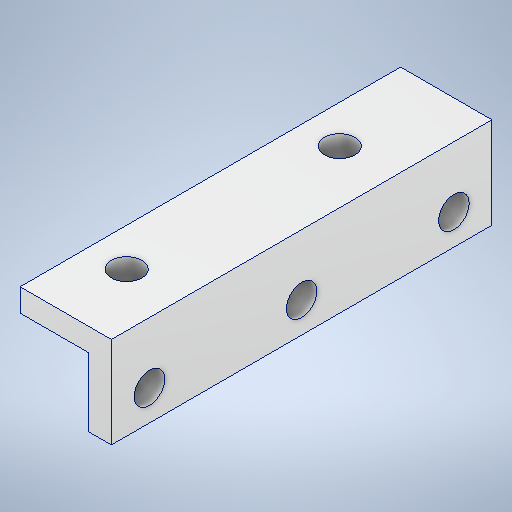
# Autodesk Inventor part: 1172
Saved by Autodesk Inventor 2025.1 (Build 291241000, 241)
## iProperties
Created: 2024-06-11
Part Number: 1172
Material: Aluminium 6061
Document SubType Name: Modeling
Designer: ffogue
Density: 2.7 g/cm^3
Appearance: Aluminium - flach
Author: ffogue
Autodesk Inventor part; units mm, degrees
ref_plane "YZ Plane" through (0, 0, 0) normal (1, 0, 0) x (0, 1, 0)
ref_plane "XZ Plane" through (0, 0, 0) normal (0, 1, 0) x (-1, 0, 0)
ref_plane "XY Plane" through (0, 0, 0) normal (0, 0, 1) x (1, 0, 0)
sketch "Skizze1" plane through (0, 0, 0) normal (0, 1, 0) x (-1, 0, 0)
  line L0 (0, 0) -> (12, 0)
  line L1 (12, 0) -> (12, -3)
  line L2 (12, -3) -> (3, -3)
  line L3 (3, -3) -> (3, -12)
  line L4 (3, -12) -> (0, -12)
  line L5 (0, -12) -> (0, 0)
  dimension "d0" = 12
  dimension "d1" = 3
  dimension "d2" = 12
  dimension "d3" = 3
  constraints: 12 end point, 5 perpendicular, 1 horizontal
  measures "d0" distance between parallel lines of L5 L1
  measures "d1" distance between parallel lines of L0 L2
  measures "d2" distance between parallel lines of L4 L0
  measures "d3" distance between parallel lines of L5 L3
extrude "Extrusion1" add sketch "Skizze1" along normal blind 50
sketch "Skizze2" plane through (-3, 0, -12) normal (-1, 0, 0) x (0, 0, 1)
  line L0 (0, 0) -> (0, 50) projected
  line L1 (12, 0) -> (0, 0) projected
  line L2 (0, 50) -> (9, 50) projected
  point P0 (4, 45)
  point P1 (4, 5)
  point P2 (0, 25)
  point P3 (4, 25)
  dimension "d13" = 4
  dimension "d29" = 5
  dimension "d30" = 5
  dimension "d31" = 20
  constraints: 2 vertical alignment, 1 midpoint
  measures "d13" distance from line of L0 point (4, 45)
  measures "d29" distance from line of L1 point (4, 5)
  measures "d30" distance from line of L2 point (4, 45)
  measures "d31" distance of point (4, 25) point (4, 5)
hole "Bohrung1" at (-3, 45, -8) at (-3, 5, -8) at (-3, 25, -8) direction (1, 0, 0) diameter 4 end through all
sketch "Skizze3" plane through (-3, 0, -3) normal (0, 0, -1) x (-1, 0, 0)
  line L0 (0, 0) -> (9, 0) projected
  line L1 (0, 50) -> (9, 50) projected
  line L2 (9, 0) -> (9, 50) projected
  point P0 (-3, 0)
  point P1 (4, 9)
  point P2 (4, 37)
  point P3 (4.5, 0)
  point P4 (9, 25)
  dimension "d26" = 28
  dimension "d28" = 5
  dimension "d32" = 9
  constraints: 2 midpoint
  measures "d26" distance of point (4, 37) point (4, 9)
  measures "d28" distance from line of L2 point (4, 9)
  measures "d32" distance from line of L0 point (4, 9)
hole "Bohrung2" at (-7, 9, -3) at (-7, 37, -3) direction (0, 0, 1) diameter 4 end through all
